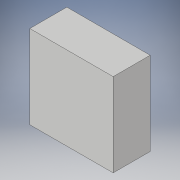
# Autodesk Inventor part: More Accurate Button Square
Saved by Autodesk Inventor 2018 (Build 220112000, 112)
## iProperties
Created: 2019-10-16
Part Number: More Accurate Button Square
Material: Generic
Document SubType Name: Modeling
Designer: Jacob
Density: 1 g/cm^3
Appearance: Default
Author: Jacob
Autodesk Inventor part; units mm, degrees
ref_plane "YZ Plane" through (0, 0, 0) normal (1, 0, 0) x (0, 1, 0)
ref_plane "XZ Plane" through (0, 0, 0) normal (0, 1, 0) x (-1, 0, 0)
ref_plane "XY Plane" through (0, 0, 0) normal (0, 0, 1) x (1, 0, 0)
sketch "Sketch1" plane through (0, 0, 0) normal (0, 0, 1) x (1, 0, 0)
  line L0 (-7.875, 7.875) -> (7.875, 7.875)
  line L1 (7.875, 7.875) -> (7.875, -7.875)
  line L2 (7.875, -7.875) -> (-7.875, -7.875)
  line L3 (-7.875, -7.875) -> (-7.875, 7.875)
  line L4 (-7.875, 7.875) -> (7.875, -7.875) construction
  line L5 (7.875, 7.875) -> (-7.875, -7.875) construction
  point P0 (0, 0)
  dimension "d0" = 15.75
  dimension "d1" = 15.75
  constraints: 12 end point, 2 midpoint, 2 parallel, 1 horizontal, 1 perpendicular
  measures "d0" distance of L0.start L0.end
  measures "d1" distance of L0.end L1.end
extrude "Extrusion1" add sketch "Sketch1" along normal blind 7
body "Solid1"
